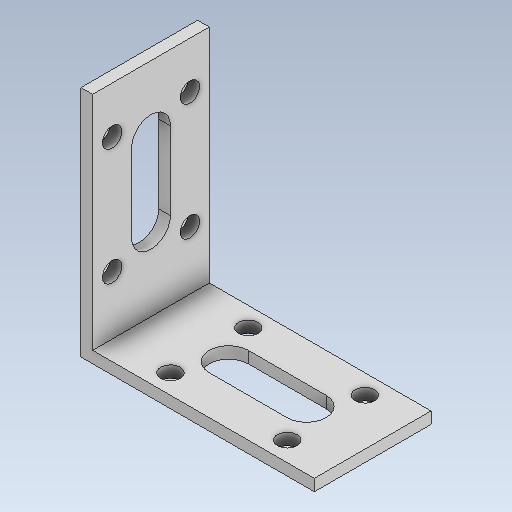
# Autodesk Inventor part: L_Bracket
Saved by Autodesk Inventor 2025.2 (Build 292293000, 293)
## iProperties
Created: 2025-05-06
Part Number: L_Bracket
Material: Generic
Document SubType Name: Modeling
Designer: Sergio Quintero
Density: 1 g/cm^3
Appearance: Default
Author: Sergio Quintero
Autodesk Inventor part; units mm, degrees
ref_plane "YZ Plane" through (0, 0, 0) normal (1, 0, 0) x (0, 1, 0)
ref_plane "XZ Plane" through (0, 0, 0) normal (0, 1, 0) x (-1, 0, 0)
sketch "Sketch1" plane through (0, 0, 0) normal (0, 1, 0) x (-1, 0, 0)
  line L0 (-30, -15) -> (30, -15)
  line L1 (30, -15) -> (30, 15)
  line L2 (30, 15) -> (-30, 15)
  line L3 (-30, 15) -> (-30, -15)
  line L4 (-30, -15) -> (30, 15) construction
  line L5 (30, -15) -> (-30, 15) construction
  point P0 (0, 0)
  dimension "d0" = 60
  dimension "d1" = 30
  constraints: 12 end point, 2 midpoint, 2 parallel, 1 horizontal, 1 perpendicular
  measures "d0" distance of L2.end L1.end
  measures "d1" distance of L1.end L0.end
extrude "Extrusion1" add sketch "Sketch1" along normal blind 3
sketch "Sketch2" plane through (0, 3, 0) normal (0, 1, 0) x (1, 0, 0)
  line L0 (-30, 15) -> (-30, -15) projected
  line L1 (30, 15) -> (-30, 15) projected
  line L2 (-30, -15) -> (-27, -15)
  line L3 (-27, -15) -> (-27, 15)
  line L4 (-27, 15) -> (-30, 15)
  line L5 (-30, 15) -> (-30, -15)
  point P0 (0, 0)
  dimension "d4" = 3
  constraints: 8 end point, 2 parallel, 1 horizontal, 1 perpendicular, 1 point on line
  measures "d4" distance of L4.end L3.end
extrude "Extrusion2" add sketch "Sketch2" along normal blind 57
sketch "Sketch3" plane through (0, 3, 0) normal (0, 1, 0) x (1, 0, 0)
  line L0 (-7, 0) -> (13, 0) construction
  line L1 (-7, -5) -> (13, -5)
  line L2 (13, 5) -> (-7, 5)
  arc A0 (-7, 5) -> (-7, -5) centre (-7, 0) ccw
  arc A1 (13, -5) -> (13, 5) centre (13, 0) ccw
  line L3 (3, 0) -> (23, 0) construction
  line L4 (-27, -15) -> (30, -15) projected
  line L5 (30, -15) -> (30, 15) projected
  circle A2 centre (18, -10) radius 2.5
  point P0 (18, 0)
  dimension "d7" = 10
  dimension "d8" = 0
  dimension "d9" = 10
  dimension "d10" = 5
  dimension "d11" = 12
  dimension "d12" = 5
  dimension "d23" = 0
  constraints: 10 end point, 5 point on circle, 4 tangent, 3 centre point, 2 horizontal, 1 coincident, 1 collinear, 1 midpoint, 1 parallel, 1 other
  measures "d7" distance of L3.start L0.end
  measures "d8" distance between parallel lines of L0 L3
  measures "d9" diameter of A1
  measures "d10" distance from line of L4 point (18, -10)
  measures "d12" diameter of A2
  measures "d23" horizontal distance of point (18, 0) A2.centre
extrude "Extrusion3" cut sketch "Sketch3" against normal through all contours A2
pattern_linear "Rectangular Pattern1" count 2 spacing 30 along (-1, 0, 0) count 2 spacing 20 along (0, 0, -1) of "Extrusion3"
extrude "Extrusion4" cut sketch "Sketch3" against normal through all contours A0 L2 A1 L1
ref_plane "Work Plane1" through (-27, 3, 0) normal (-0.7071, 0.7071, 0) x (0, 0, 1)
mirror "Mirror1" about plane through (-27, 3, 0) normal (-0.7071, 0.7071, 0) of "Extrusion3", "Rectangular Pattern1", "Extrusion4"
body "Solid1"
